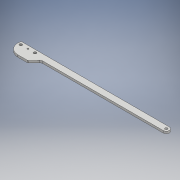
# Autodesk Inventor part: poweredArm
Saved by Autodesk Inventor 2018 (Build 220112000, 112)
## iProperties
Created: 2017-12-31
Part Number: poweredArm
Material: Generic
Document SubType Name: Modeling
Designer: mzhang
Density: 1 g/cm^3
Appearance: Default
Author: mzhang
Autodesk Inventor part; units mm, degrees
ref_plane "YZ Plane" through (0, 0, 0) normal (1, 0, 0) x (0, 1, 0)
ref_plane "XZ Plane" through (0, 0, 0) normal (0, 1, 0) x (-1, 0, 0)
ref_plane "XY Plane" through (0, 0, 0) normal (0, 0, 1) x (1, 0, 0)
sketch "Sketch1" plane through (0, 0, 0) normal (0, 0, 1) x (1, 0, 0)
  arc A0 (13.7445, 2.5) -> (13.7445, -2.5) centre (0, 0) ccw
  circle A1 centre (-9.779, 0) radius 1.8415
  circle A2 centre (9.779, 0) radius 1.8415
  line L0 (190.5, -2.5) -> (13.7445, -2.5)
  line L1 (13.7445, -2.5) -> (13.7445, 2.5)
  line L2 (13.7445, 2.5) -> (190.5, 2.5)
  line L3 (190.5, 2.5) -> (190.5, -2.5)
  line L4 (190.5, -2.5) -> (13.7445, 2.5) construction
  line L5 (13.7445, -2.5) -> (190.5, 2.5) construction
  line L6 (0, 13.97) -> (13.7445, 13.97)
  line L7 (0, -13.97) -> (13.7445, -13.97)
  line L8 (13.7445, -13.97) -> (24.8209, -2.5)
  line L9 (13.7445, 13.97) -> (24.8209, 2.5)
  point P0 (102.1222, 0)
  dimension "d0" = 27.94
  dimension "d1" = 3.683
  dimension "d2" = 3.683
  dimension "d3" = 5
  dimension "d5" = 134
  dimension "d19" = 190.5
  constraints: 20 end point, 4 point on circle, 3 centre point, 3 parallel, 2 horizontal, 2 midpoint, 2 point on line, 1 coincident, 1 perpendicular, 1 tangent
  measures "d0" diameter of A0
  measures "d1" diameter of A1
  measures "d2" diameter of A2
  measures "d3" distance of L0.end L1.end
  measures "d5" angle of L8 L7
  measures "d19" distance from line of L3 point (0, 0)
extrude "Extrusion1" add sketch "Sketch1" along normal blind 3
fillet "Fillet1" radius 2 4 edges at (13.7445, -13.97, 1.5) (13.7445, 13.97, 1.5) (24.8209, 2.5, 1.5) (24.8209, -2.5, 1.5)
sketch "Sketch2" plane through (0, 0, 3) normal (0, 0, 1) x (1, 0, 0)
  line L0 (190.5, -2.5) -> (190.5, 2.5) projected
  circle A0 centre (190.5, 0) radius 4.25
  circle A1 centre (190.5, 0) radius 1.778
  point P0 (0, 0)
  dimension "d9" = 8.5
  dimension "d23" = 3.556
  dimension "d26" = 0
  constraints: 2 centre point, 1 coincident
  measures "d9" diameter of A0
  measures "d23" diameter of A1
  measures "d26" distance from line of L0 A0.centre
extrude "Extrusion2" add sketch "Sketch2" against normal up to surface (3 mm away)
extrude "Extrusion3" cut sketch "Sketch2" against normal up to surface (3 mm away) contours A1 L0 | L0 A1
extrude "Extrusion4" add sketch "Sketch2" along normal mid plane 6 contours A1 L0 | L0 A1
sketch "Sketch3" plane through (0, 0, 3) normal (0, 0, 1) x (1, 0, 0)
  circle A0 centre (0, 0) radius 1
  dimension "d16" = 2
  constraints: 1 centre point, 1 coincident
  measures "d16" diameter of A0
extrude "Extrusion5" cut sketch "Sketch3" against normal up to surface (3 mm away)
sketch "Sketch4" plane through (0, 0, 0) normal (0, 0, -1) x (-1, 0, 0)
  arc A0 (-187.0631, 2.5) -> (-187.0631, -2.5) centre (-190.5, 0) ccw projected
  line L0 (-190.5, -4.25) -> (-23.131, -4.25)
  line L1 (-14.3342, -13.3593) -> (-24.2312, -3.1107) projected
  line L2 (-24.2312, 3.1107) -> (-14.3342, 13.3593) projected
  line L3 (-23.131, 4.25) -> (-190.5, 4.25)
  line L4 (-25.6699, -2.5) -> (-187.0631, -2.5) projected
  arc A1 (-24.2312, -3.1107) -> (-25.6699, -2.5) centre (-25.6699, -4.5) ccw projected
  arc A2 (-25.6699, 2.5) -> (-24.2312, 3.1107) centre (-25.6699, 4.5) ccw projected
  line L5 (-187.0631, 2.5) -> (-25.6699, 2.5) projected
  point P0 (0, 0)
  point P1 (-190.5, -2.5)
  point P2 (-190.5, 2.5)
  constraints: 4 end point, 2 horizontal, 2 point on circle, 2 point on line
extrude "Extrusion6" add sketch "Sketch4" against normal up to surface (3 mm away)
fillet "Fillet2" radius 4 2 edges at (23.131, -4.25, 1.5) (23.131, 4.25, 1.5)
sketch "Sketch5" plane through (190.5, 0, 6) normal (0, 0, 1) x (1, 0, 0)
  circle A0 centre (0, 0) radius 1.778 projected
  point P0 (-190.5, 0)
extrude "Extrusion7" cut sketch "Sketch5" against normal up to surface (6 mm away)
sketch "Sketch6" plane through (0, 0, 3) normal (0, 0, 1) x (1, 0, 0)
  line L0 (24.8289, 4.25) -> (190.5, 4.25) projected
  line L1 (24.8289, 4.25) -> (-13.722, 4.25)
  arc A0 (21.9515, 5.4714) -> (24.8289, 4.25) centre (24.8289, 8.25) ccw projected
  line L2 (-13.722, 4.25) -> (-32.1896, 106.8935)
  line L3 (-32.1896, 106.8935) -> (179.5248, 4.25)
  line L4 (179.5248, 4.25) -> (-13.722, 4.25)
  point P0 (0, 0)
  constraints: 8 end point, 3 point on line, 2 horizontal, 1 tangent
extrude "Extrusion8" cut sketch "Sketch6" against normal up to surface (3 mm away)
body "Solid1"
